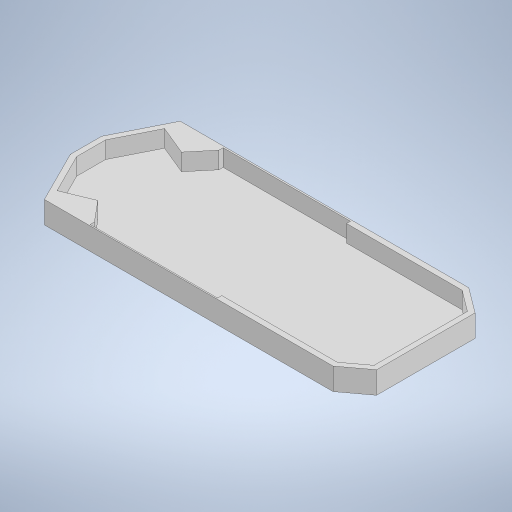
# Autodesk Inventor part: h6-case
Saved by Autodesk Inventor 2024.1 (Build 281209000, 209)
## iProperties
Created: 2025-08-18
Part Number: h6-case
Material: Generic
Document SubType Name: Modeling
Designer: iwheard
Density: 1 g/cm^3
Appearance: Default
Author: iwheard
Autodesk Inventor part; units mm, degrees
ref_plane "YZ Plane" through (0, 0, 0) normal (1, 0, 0) x (0, 1, 0)
ref_plane "XZ Plane" through (0, 0, 0) normal (0, 1, 0) x (-1, 0, 0)
ref_plane "XY Plane" through (0, 0, 0) normal (0, 0, 1) x (1, 0, 0)
sketch "Sketch1" plane through (0, 0, 0) normal (0, 1, 0) x (-1, 0, 0)
  line L0 (-197, -67.45) -> (-197, -12.45)
  line L1 (-3, -31.35) -> (-3, -48.35)
  line L2 (-200, -79.9) -> (0, -79.9)
  line L3 (0, -79.9) -> (0, 0)
  line L4 (0, 0) -> (-200, 0)
  line L5 (-200, 0) -> (-200, -79.9)
  line L6 (-184.6, -76.7) -> (-197, -67.45)
  line L7 (-184.6, -3.2) -> (-197, -12.45)
  line L8 (-184.6, -76.7) -> (-116.6, -76.7)
  line L9 (-184.6, -3.2) -> (-116.6, -3.2)
  line L10 (-41.6, -3.2) -> (-41.6, -0.7)
  line L11 (-41.6, -0.7) -> (-116.6, -0.7)
  line L12 (-116.6, -0.7) -> (-116.6, -3.2)
  line L13 (-41.6, -76.5) -> (-41.6, -79)
  line L14 (-41.6, -79) -> (-116.6, -79)
  line L15 (-116.6, -79) -> (-116.6, -76.7)
  line L16 (-3, -31.35) -> (-3, -48.35)
  line L17 (-3, -48.35) -> (-14.6, -71.5)
  line L18 (-31.6, -64.5) -> (-41.6, -76.5)
  line L19 (-3, -31.35) -> (-14.6, -8.2)
  line L20 (-14.6, -8.2) -> (-31.6, -15.2)
  line L21 (-31.6, -15.2) -> (-41.6, -3.2)
  line L22 (-31.6, -64.5) -> (-14.6, -71.5)
  point P0 (-197, 35.2625)
  point P1 (-197, -38.4375)
  dimension "d2" = 194
  dimension "d8" = 55
  dimension "d14" = 73.5
  dimension "d20" = 75
  dimension "d21" = 10
  dimension "d22" = 17
  dimension "d24" = 7
  dimension "d25" = 17
  dimension "d29" = 7
  dimension "d30" = 3
  dimension "d31" = 3
  dimension "d32" = 23.15
  dimension "d33" = 23.15
  dimension "d34" = 12
  dimension "d35" = 12
  dimension "d36" = 2.5
  dimension "d38" = 3.2
  dimension "d39" = 3.2
  dimension "d40" = 12.4
  dimension "d41" = 9.25
  dimension "d42" = 68
  dimension "d43" = 2.5
  dimension "d50" = 9.25
  dimension "d51" = 155.4
  constraints: 46 end point, 14 vertical alignment, 5 horizontal alignment, 2 coincident
  measures "d2" distance between parallel lines of L0 L1
  measures "d8" distance of L0.start L0.end
  measures "d14" distance between parallel lines of L9 L8
  measures "d20" distance between parallel lines of L12 L10
  measures "d21" horizontal distance of L10.start L20.end
  measures "d22" horizontal distance of L19.end L20.end
  measures "d24" vertical distance of L19.end L20.end
  measures "d25" distance of L1.start L1.end
  measures "d29" vertical distance of L18.start L17.end
  measures "d30" distance between parallel lines of L5 L0
  measures "d31" distance between parallel lines of L1 L3
  measures "d32" vertical distance of L1.start L19.end
  measures "d33" vertical distance of L17.end L1.end
  measures "d34" vertical distance of L18.start L13.start
  measures "d35" vertical distance of L10.start L20.end
  measures "d36" distance of L13.start L13.end
  measures "d38" distance between parallel lines of L4 L9
  measures "d39" distance between parallel lines of L8 L2
  measures "d40" horizontal distance of L0.start L6.start
  measures "d41" distance from line of L0.start L8
  measures "d42" distance from line of L6.start L15
  measures "d43" distance between parallel lines of L11 L9
  measures "d50" vertical distance of L0.end L7.start
  measures "d51" distance from line of L10.start L0
extrude "Extrusion1" add sketch "Sketch1" along normal blind 10
sketch "Sketch2" plane through (0, 0, 0) normal (0, -1, 0) x (1, 0, 0)
  line L0 (0, -79.9) -> (0, 0) projected
  line L1 (200, -79.9) -> (0, -79.9) projected
  line L2 (200, 0) -> (200, -79.9) projected
  line L3 (0, 0) -> (200, 0) projected
extrude "Extrusion2" add sketch "Sketch2" along normal blind 3
sketch "Sketch3" plane through (0, 10, 0) normal (0, 1, 0) x (1, 0, 0)
  line L0 (17.8016, -4.8861) -> (-9.7741, 50.1464)
  line L1 (-8.7292, 31.6387) -> (22.6961, 94.354)
  line L2 (0, 79.9) -> (0, 0) projected
  line L3 (0, 0) -> (200, 0) projected
  line L4 (200, 0) -> (200, 79.9) projected
  line L5 (200, 79.9) -> (0, 79.9) projected
  line L6 (14.6, 8.2) -> (3, 31.35) projected
  line L7 (3, 31.35) -> (3, 48.35) projected
  line L8 (3, 48.35) -> (14.6, 71.5) projected
  line L9 (14.6, 71.5) -> (31.6, 64.5) projected
  line L10 (31.6, 64.5) -> (41.6, 76.5) projected
  line L11 (41.6, 76.5) -> (41.6, 79) projected
  line L12 (41.6, 79) -> (116.6, 79) projected
  line L13 (116.6, 79) -> (116.6, 76.7) projected
  line L14 (116.6, 76.7) -> (184.6, 76.7) projected
  line L15 (184.6, 76.7) -> (197, 67.45) projected
  line L16 (197, 67.45) -> (197, 12.45) projected
  line L17 (197, 12.45) -> (184.6, 3.2) projected
  line L18 (184.6, 3.2) -> (116.6, 3.2) projected
  line L19 (116.6, 3.2) -> (116.6, 0.7) projected
  line L20 (116.6, 0.7) -> (41.6, 0.7) projected
  line L21 (41.6, 0.7) -> (41.6, 3.2) projected
  line L22 (41.6, 3.2) -> (31.6, 15.2) projected
  line L23 (31.6, 15.2) -> (14.6, 8.2) projected
  line L24 (14.6, 8.2) -> (3, 31.35) projected
  line L25 (185.0423, 80.1128) -> (210.2776, 61.2881)
  line L26 (215.6714, 68) -> (215.6714, 11.7)
  line L27 (210.454, 18.7435) -> (184.2237, -0.8235)
  line L28 (184.6, 76.7) -> (197, 67.45) projected
  point P0 (185.3276, 79.9)
  point P1 (200, 68.9549)
  point P2 (200, 10.9451)
  point P3 (185.3276, 0)
  point P4 (15.3533, 0)
  point P5 (0, 30.6404)
  point P6 (15.4535, 79.9)
  point P7 (0, 49.0596)
  dimension "d44" = 3
  dimension "d45" = 3
  dimension "d46" = 3
  dimension "d47" = 3
  constraints: 10 end point, 4 parallel
  measures "d44" distance between parallel lines of L1 L8
  measures "d45" distance between parallel lines of L0 L6
  measures "d46" distance between parallel lines of L25 L15
  measures "d47" distance between parallel lines of L17 L27
extrude "Extrusion3" cut sketch "Sketch3" against normal through all contours L3 L2 L0 | L27 L4 L3 | L2 L5 L1 | L25 L5 L4
body "Solid1"
